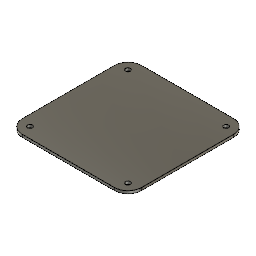
Front_pannel v1 (Autodesk Fusion 360 design; units mm, degrees)
Autodesk Fusion 360 part; units mm, degrees
sketch "Sketch1" plane through (0, 0, 0) normal (0, 0, 1) x (1, 0, 0)
  line L0 (43.25, 43.25) -> (-43.25, 43.25)
  line L1 (-43.25, 43.25) -> (-43.25, -43.25)
  line L2 (-43.25, -43.25) -> (43.25, -43.25)
  line L3 (43.25, -43.25) -> (43.25, 43.25)
  line L4 (43.25, 43.25) -> (-43.25, -43.25) construction
  line L5 (-43.25, 43.25) -> (43.25, -43.25) construction
  dimension "d17" = 86.5
  dimension "d18" = 86.5
  measures "d17" distance of L1.end L2.end
  measures "d18" distance of L0.end L1.end
extrude "Extrude1" add sketch "Sketch1" along normal blind 2
fillet "Fillet1" radius 10 1 edges at (-43.25, -43.25, 1)
fillet "Fillet2" radius 10 1 edges at (43.25, -43.25, 1)
fillet "Fillet3" radius 10 1 edges at (43.25, 43.25, 1)
fillet "Fillet4" radius 10 1 edges at (-43.25, 43.25, 1)
sketch "Sketch2" plane through (0, 0, 2) normal (0, 0, 1) x (-1, 0, 0)
  arc A0 (33.25, -43.25) -> (43.25, -33.25) centre (33.25, -33.25) ccw
  line L0 (43.25, -33.25) -> (43.25, 33.25)
  arc A1 (43.25, 33.25) -> (33.25, 43.25) centre (33.25, 33.25) ccw
  line L1 (33.25, 43.25) -> (-33.25, 43.25)
  arc A2 (-33.25, 43.25) -> (-43.25, 33.25) centre (-33.25, 33.25) ccw
  line L2 (-43.25, 33.25) -> (-43.25, -33.25)
  arc A3 (-43.25, -33.25) -> (-33.25, -43.25) centre (-33.25, -33.25) ccw
  line L3 (-33.25, -43.25) -> (33.25, -43.25)
  point P0 (35.5, -35.5)
  point P1 (-35.5, -35.5)
  point P2 (-35.5, 35.5)
  point P3 (35.5, 35.5)
  dimension "d25" = 35.5
  dimension "d26" = 35.5
  dimension "d27" = 71
  dimension "d28" = 71
  measures "d25" distance of origin P1
  measures "d26" distance of origin P1
  measures "d27" distance of P0 P1
  measures "d28" distance of P1 P2
hole "Hole1" at (-35.5, 35.5, 2) at (35.5, 35.5, 2) at (35.5, -35.5, 2) at (-35.5, -35.5, 2) direction (0, 0, -1) diameter 3.5 depth 30 tip angle 118
